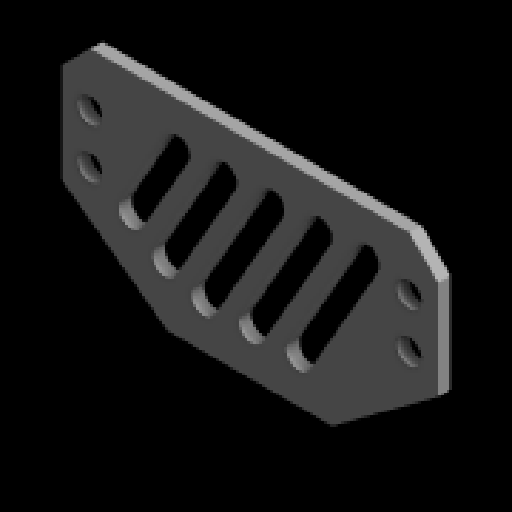
# Autodesk Inventor part: NoseMount
Saved by Autodesk Inventor 2025.2 (Build 292293000, 293)
## iProperties
Created: 2024-12-21
Part Number: NoseMount
Material: Generic
Document SubType Name: Sheet Metal
Designer: valer
Density: 1 g/cm^3
Sheet Metal Rule: Default
Appearance: Default
Author: valer
Autodesk Inventor part; units mm, degrees
ref_plane "YZ Plane" through (0, 0, 0) normal (1, 0, 0) x (0, 1, 0)
ref_plane "XZ Plane" through (0, 0, 0) normal (0, 1, 0) x (-1, 0, 0)
ref_plane "XY Plane" through (0, 0, 0) normal (0, 0, 1) x (1, 0, 0)
sketch "Sketch1" plane through (0, 0, 0) normal (0, 0, 1) x (1, 0, 0)
  circle A0 centre (11, 6) radius 2.7 construction
  circle A1 centre (11, -6) radius 2.7 construction
  line L0 (49.7615, -342.4426) -> (49.7615, 314.6303) construction
  line L1 (11, 12) -> (-4.4335, 12) construction
  line L2 (-17, -12) -> (11, -12) construction
  line L3 (4, 12) -> (4, -12)
  line L4 (4, 12) -> (11, 19)
  line L5 (11, 19) -> (49.7615, 19)
  line L6 (19.0192, 2.5843) -> (28.2364, 13.6384) construction
  circle A2 centre (11, 6) radius 3
  circle A3 centre (11, -6) radius 3
  circle A4 centre (88.5231, 6) radius 3
  circle A5 centre (88.5231, -6) radius 3
  line L7 (4, -12) -> (29.7615, -31)
  line L8 (29.7615, -31) -> (49.7615, -31)
  line L9 (95.5231, 12) -> (95.5231, -12)
  line L10 (95.5231, 12) -> (88.5231, 19)
  line L11 (88.5231, 19) -> (49.7615, 19)
  line L12 (95.5231, -12) -> (69.7615, -31)
  line L13 (69.7615, -31) -> (49.7615, -31)
  point P0 (0, 0)
  dimension "d0" = 7
  dimension "d6" = 6
  dimension "d7" = 6
  dimension "d14" = 7
  dimension "d15" = 50
  dimension "d16" = 20
  dimension "d38" = 135
  measures "d0" distance from line of A0.centre L3
  measures "d6" diameter of A2
  measures "d7" diameter of A3
  measures "d14" distance between parallel lines of L5 L1
  measures "d15" distance between parallel lines of L8 L5
  measures "d16" distance of L7.end L8.end
  measures "d38" angle of L5 L4
extrude "Plate1" add sketch "Sketch1" along normal blind 3
sketch "Sketch5" plane through (0, 0, 3) normal (0, 0, 1) x (1, 0, 0)
  circle A0 centre (88.5231, -6) radius 3 construction
  line L0 (4, -12) -> (4, 12) construction
  line L1 (29.7615, -31) -> (4, -12) construction
  line L2 (69.7615, -31) -> (29.7615, -31) construction
  line L3 (95.5231, -12) -> (69.7615, -31) construction
  line L4 (95.5231, 12) -> (95.5231, -12) construction
  line L5 (88.5231, 19) -> (95.5231, 12) construction
  line L6 (11, 19) -> (88.5231, 19) construction
  line L7 (4, 12) -> (11, 19) construction
  line L8 (85.2094, 11) -> (87.5231, 8.6863) construction
  line L9 (87.5231, 8.6863) -> (87.5231, -7.9598) construction
  line L10 (87.5231, -7.9598) -> (67.1305, -23) construction
  line L11 (67.1305, -23) -> (32.3926, -23) construction
  line L12 (32.3926, -23) -> (12, -7.9598) construction
  line L13 (12, -7.9598) -> (12, 8.6863) construction
  line L14 (12, 8.6863) -> (14.3137, 11) construction
  line L15 (14.3137, 11) -> (85.2094, 11) construction
  line L16 (18, 11) -> (18, -12.385) construction
  line L17 (49.7615, 11) -> (49.7615, -23) construction
  line L18 (81.5231, 11) -> (81.5231, -12.385) construction
  line L19 (33.6401, 11) -> (19.5, -13.4913) construction
  line L20 (29.542, 9.9019) -> (18.4019, -9.3932)
  line L21 (23.5981, -12.3932) -> (34.7381, 6.9019)
  arc A1 (34.7381, 6.9019) -> (29.542, 9.9019) centre (32.1401, 8.4019) ccw
  arc A2 (18.4019, -9.3932) -> (23.5981, -12.3932) centre (21, -10.8932) ccw
  line L22 (45.1871, 11) -> (27.5985, -19.4642) construction
  line L23 (41.089, 9.9019) -> (26.5005, -15.3662)
  line L24 (31.6966, -18.3662) -> (46.2851, 6.9019)
  arc A3 (46.2851, 6.9019) -> (41.089, 9.9019) centre (43.6871, 8.4019) ccw
  arc A4 (26.5005, -15.3662) -> (31.6966, -18.3662) centre (29.0985, -16.8662) ccw
  line L25 (56.7341, 11) -> (37.1042, -23) construction
  line L26 (52.636, 9.9019) -> (36.0061, -18.9019)
  line L27 (41.2022, -21.9019) -> (57.8321, 6.9019)
  arc A5 (57.8321, 6.9019) -> (52.636, 9.9019) centre (55.2341, 8.4019) ccw
  arc A6 (36.0061, -18.9019) -> (41.2022, -21.9019) centre (38.6042, -20.4019) ccw
  line L28 (68.2811, 11) -> (48.6512, -23) construction
  line L29 (64.183, 9.9019) -> (47.5531, -18.9019)
  line L30 (52.7492, -21.9019) -> (69.3791, 6.9019)
  arc A7 (69.3791, 6.9019) -> (64.183, 9.9019) centre (66.7811, 8.4019) ccw
  arc A8 (47.5531, -18.9019) -> (52.7492, -21.9019) centre (50.1512, -20.4019) ccw
  line L31 (79.8281, 11) -> (60.1982, -23) construction
  line L32 (75.73, 9.9019) -> (59.1001, -18.9019)
  line L33 (64.2962, -21.9019) -> (80.9262, 6.9019)
  arc A9 (80.9262, 6.9019) -> (75.73, 9.9019) centre (78.3281, 8.4019) ccw
  arc A10 (59.1001, -18.9019) -> (64.2962, -21.9019) centre (61.6982, -20.4019) ccw
  point P0 (26.57, -1.2456)
  point P1 (36.3928, -4.2321)
  point P2 (46.9191, -6)
  point P3 (58.4661, -6)
  point P4 (70.0131, -6)
  dimension "d61" = 8
  dimension "d62" = 14
  dimension "d63" = 3
  dimension "d64" = 60
  dimension "d65" = 4
  dimension "d66" = 4
  dimension "d67" = 4
  dimension "d68" = 4
  constraints: 60 end point, 30 point on circle, 21 tangent, 16 point on line, 12 centre point, 9 parallel, 6 midpoint, 4 equal radius, 2 symmetric about line, 1 vertical, 17 other
  measures "d62" distance between parallel lines of L0 L16
  measures "d63" radius of A1
  measures "d64" angle to the sketch x axis of L19
  measures "d65" distance between parallel lines of L23 L21
  measures "d66" distance between parallel lines of L26 L24
  measures "d67" distance between parallel lines of L29 L27
  measures "d68" distance between parallel lines of L32 L30
extrude "Cut2" cut sketch "Sketch5" against normal blind 3
equation "\"d9\" = Thickness"
equation "\"BendRadius\" = Thickness"
equation "\"BendReliefWidth\" = Thickness"
equation "\"BendReliefDepth\" = 0.5 * Thickness"
equation "\"CornerReliefSize\" = 4 * Thickness"
equation "\"MinimumRemnant\" = 2 * Thickness"
equation "\"TransitionRadius\" = BendRadius"
equation "\"JacobiRadiusSize\" = BendRadius"
equation "\"GapSize\" = Thickness"
equation "\"Thickness\" = 3"
body "Solid1"
